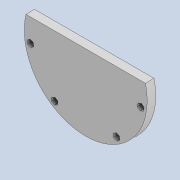
# Autodesk Inventor part: plate_third_floor
Saved by Autodesk Inventor 2020.4 (Build 244396000, 396)
## iProperties
Created: 2021-05-05
Part Number: plate_third_floor
Material: Generic
Document SubType Name: Modeling
Designer: Acer
Density: 1 g/cm^3
Appearance: Default
Author: Acer
Autodesk Inventor part; units mm, degrees
ref_plane "YZ Plane" through (0, 0, 0) normal (1, 0, 0) x (0, 1, 0)
ref_plane "XZ Plane" through (0, 0, 0) normal (0, 1, 0) x (-1, 0, 0)
ref_plane "XY Plane" through (0, 0, 0) normal (0, 0, 1) x (1, 0, 0)
sketch "Sketch1" plane through (0, 0, 0) normal (0, 0, 1) x (1, 0, 0)
  circle A0 centre (0, 0) radius 85.8
  line L0 (-72.5268, -13.7582) -> (-76.3217, -16.8148)
  line L1 (-76.3217, -16.8148) -> (-80.8663, -15.0566)
  line L2 (-80.8663, -15.0566) -> (-81.616, -10.2418)
  line L3 (-81.616, -10.2418) -> (-77.8211, -7.1852)
  line L4 (-77.8211, -7.1852) -> (-73.2765, -8.9434)
  line L5 (-73.2765, -8.9434) -> (-72.5268, -13.7582)
  line L6 (73.2765, -8.9434) -> (77.8211, -7.1852)
  line L7 (77.8211, -7.1852) -> (81.616, -10.2418)
  line L8 (81.616, -10.2418) -> (80.8663, -15.0566)
  line L9 (80.8663, -15.0566) -> (76.3217, -16.8148)
  line L10 (76.3217, -16.8148) -> (72.5268, -13.7582)
  line L11 (72.5268, -13.7582) -> (73.2765, -8.9434)
  line L12 (-77.0714, -12) -> (0, 0) construction
  line L13 (77.0714, -12) -> (0, 0) construction
  line L14 (0, 0) -> (85.8, 0) construction
  line L15 (47.5879, -67.0929) -> (43.5316, -69.793)
  line L16 (47.2777, -62.2299) -> (47.5879, -67.0929)
  line L17 (42.9111, -60.0671) -> (47.2777, -62.2299)
  line L18 (38.8548, -62.7673) -> (42.9111, -60.0671)
  line L19 (39.165, -67.6302) -> (38.8548, -62.7673)
  line L20 (43.5316, -69.793) -> (39.165, -67.6302)
  line L21 (-47.2777, -62.2299) -> (-42.9111, -60.0671)
  line L22 (-42.9111, -60.0671) -> (-38.8548, -62.7673)
  line L23 (-38.8548, -62.7673) -> (-39.165, -67.6302)
  line L24 (-39.165, -67.6302) -> (-43.5316, -69.793)
  line L25 (-43.5316, -69.793) -> (-47.5879, -67.0929)
  line L26 (-47.5879, -67.0929) -> (-47.2777, -62.2299)
  line L27 (-83.4364, 20) -> (83.4364, 20)
  point P0 (43.2214, -64.9301)
  point P1 (-43.2214, -64.9301)
  dimension "d0" = 171.6
  dimension "d1" = 78
  dimension "d2" = 78
  dimension "d5" = 12
  dimension "d6" = 4.22
  dimension "d7" = 4.22
  dimension "d10" = 12
  dimension "d13" = 47.5
  dimension "d17" = 47.5
  dimension "d19" = 20
  constraints: 56 end point, 3 point on circle, 2 horizontal, 2 perpendicular, 1 centre point, 1 coincident, 54 other
  measures "d0" diameter of A0
  measures "d1" distance of L12.start point (0, 0)
  measures "d2" distance of point (0, 0) L13.start
  measures "d5" distance from line of L14 L13.start
  measures "d6" distance from line of L13.start L11
  measures "d7" distance from line of L5 L12.start
  measures "d10" vertical distance of point (0, 0) L12.start
  measures "d19" distance from line of L27 L12.end
extrude "Extrusion1" add sketch "Sketch1" against normal blind 12 contours A0 L27 picked at (-14.3037, -29.1945)
body "Solid1"
